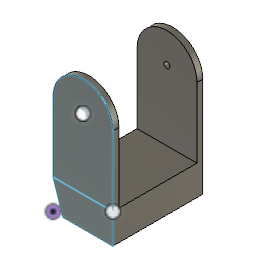
robosoc_legs_holder (Autodesk Fusion 360 design; units mm, degrees)
part number: 2025-12-04-10-49-25-755
Autodesk Fusion 360 part; units mm, degrees
sketch "Sketch1" plane through (0, 0, 0) normal (0, 1, 0) x (1, 0, 0)
  line L0 (5, 0) -> (30, 0)
  line L1 (30, 0) -> (30, -50)
  line L2 (0, -50) -> (0, -15)
  arc A0 (0, -50) -> (30, -50) centre (15, -50) ccw
  circle A1 centre (15, -50) radius 1.5
  line L3 (30, 0) -> (5, 0) construction
  line L4 (0, -15) -> (5, 0)
  line L5 (0, -15) -> (30, -15)
  dimension "d2" = 50
  dimension "d4" = 3
  dimension "d5" = 25
  dimension "d6" = 15
  dimension "d9" = 30
  constraint horizontal L0
  constraint vertical L1
  constraint vertical L2
  constraint concentric A0 A1
  constraint perpendicular L1 L3
  constraint perpendicular L1 L5
  measures "d2" distance of origin L2.start
  measures "d4" diameter of A1
  measures "d5" distance of L0.end L0.start
  measures "d6" distance of origin L2.end
  measures "d9" distance of L2.end L5.end
extrude "Extrude1" add sketch "Sketch1" along normal blind 3
extrude "Extrude2" cut sketch "Sketch1" along normal blind 45 contours L0 L1 L4 L5
extrude "Extrude3" add sketch "Sketch1" along normal blind 22.5 contours L0 L1 L4 L5
mirror "Mirror1" about plane through (0, 22.5, 0) normal (0, 1, 0) of bodies 1 merged
hole "Hole1" at (17.5, 22.5, 0) direction (0, 0, 1) diameter 20 depth 13 tip angle 180
